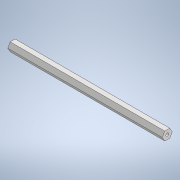
# Autodesk Inventor part: 5mm hex shaft
Saved by Autodesk Inventor 2022 (Build 260153000, 153)
## iProperties
Created: 2022-04-17
Part Number: 5mm hex shaft
Material: Generic
Document SubType Name: Modeling
Designer: matt
Density: 1 g/cm^3
Appearance: Default
Author: matt
Autodesk Inventor part; units mm, degrees
ref_plane "YZ Plane" through (0, 0, 0) normal (1, 0, 0) x (0, 1, 0)
ref_plane "XZ Plane" through (0, 0, 0) normal (0, 1, 0) x (-1, 0, 0)
ref_plane "XY Plane" through (0, 0, 0) normal (0, 0, 1) x (1, 0, 0)
sketch "Sketch1" plane through (0, 0, 0) normal (1, 0, 0) x (0, 1, 0)
  line L0 (0, -2.8868) -> (-2.5, -1.4434)
  line L1 (-2.5, -1.4434) -> (-2.5, 1.4434)
  line L2 (-2.5, 1.4434) -> (0, 2.8868)
  line L3 (0, 2.8868) -> (2.5, 1.4434)
  line L4 (2.5, 1.4434) -> (2.5, -1.4434)
  line L5 (2.5, -1.4434) -> (0, -2.8868)
  circle A0 centre (0, 0) radius 0.8728
  dimension "d0" = 5
  constraints: 12 end point, 2 coincident, 1 centre point, 13 other
  measures "d0" distance between parallel lines of L1 L4
extrude "Extrusion1" add sketch "Sketch1" along normal blind 89.785
body "Solid1"
